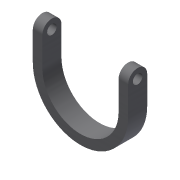
# Autodesk Inventor part: Forl
Saved by Autodesk Inventor 2022 Beta2 (Build 260130000, 130) ContinuousBuild 0
## iProperties
Created: 2008-03-12
Part Number: Forl
Document SubType Name: Modeling
Designer: jmacmillan
Density: 1 g/cm^3
Material: Generic
Appearance: Light Gray
Author: jmacmillan
Autodesk Inventor part; units mm, degrees
ref_plane "YZ Plane" through (0, 0, 0) normal (1, 0, 0) x (0, 1, 0)
ref_plane "XZ Plane" through (0, 0, 0) normal (0, 1, 0) x (-1, 0, 0)
ref_plane "XY Plane" through (0, 0, 0) normal (0, 0, 1) x (1, 0, 0)
sketch "Sketch1" plane through (0, 0, 0) normal (0, 0, 1) x (1, 0, 0)
  line L0 (-101.6, 101.6) -> (-101.6, 0)
  arc A0 (-101.6, 0) -> (101.6, 0) centre (0, 0) ccw
  line L1 (101.6, 0) -> (101.6, 101.6)
  line L2 (-127, 101.6) -> (-127, 0)
  arc A1 (-127, 0) -> (127, 0) centre (0, 0) ccw
  line L3 (127, 0) -> (127, 101.6)
  line L4 (-127, 101.6) -> (-101.6, 101.6)
  line L5 (101.6, 101.6) -> (127, 101.6)
  dimension "d0" = 101.6
  dimension "d1" = 101.6
  dimension "d2" = 25.4
  constraints: 12 end point, 4 point on circle, 3 equal length, 2 centre point, 2 tangent, 1 coincident, 1 parallel, 1 perpendicular, 1 vertical, 2 other
  measures "d0" distance of L0.start L0.end
  measures "d1" radius of A0
  measures "d2" distance between parallel lines of L2 L0
extrude "Extrusion1" add sketch "Sketch1" along normal mid plane 50.8
full round fillet "Fillet1" first side at (-110.0667, 33.8667, 25.4) centre faces at (110.0667, 101.6, -8.4667) second side at (-110.0667, 33.8667, -25.4)
full round fillet "Fillet2" first side at (-118.5333, 33.8667, 25.4) centre faces at (-118.5333, 101.6, 8.4667) second side at (-118.5333, 33.8667, -25.4)
hole "Hole1" at (127, 76.2, 0) direction (-1, 0, 0) diameter 25.4 end through all
body "Solid1"
